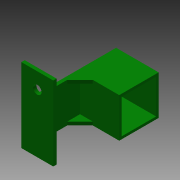
# Autodesk Inventor part: cameraMount
Saved by Autodesk Inventor 2014 (Build 180170000, 170)
## iProperties
Created: 2014-03-23
Part Number: cameraMount
Material: Generic
Document SubType Name: Modeling
Designer: jferner
Density: 1 g/cm^3
Appearance: Dark Green
Author: jferner
Autodesk Inventor part; units mm, degrees
ref_plane "YZ Plane" through (0, 0, 0) normal (1, 0, 0) x (0, 1, 0)
ref_plane "XZ Plane" through (0, 0, 0) normal (0, 1, 0) x (-1, 0, 0)
ref_plane "XY Plane" through (0, 0, 0) normal (0, 0, 1) x (1, 0, 0)
sketch "Sketch2" plane through (0, 0, 0) normal (1, 0, 0) x (0, 1, 0)
  line L0 (0, 0) -> (23.55, 0)
  line L1 (23.55, 0) -> (23.55, 23.55)
  line L2 (23.55, 23.55) -> (0, 23.55)
  line L3 (0, 23.55) -> (0, 0)
  line L4 (1.5, 1.5) -> (22.05, 1.5)
  line L5 (22.05, 1.5) -> (22.05, 22.05)
  line L6 (22.05, 22.05) -> (1.5, 22.05)
  line L7 (1.5, 22.05) -> (1.5, 1.5)
  dimension "d0" = 1.5
  dimension "d1" = 1.5
  dimension "d2" = 1.5
  dimension "d3" = 1.5
  dimension "d4" = 20.55
  dimension "d5" = 20.55
  dimension "widthSqAlum" = 23.55
  constraints: 16 end point, 4 parallel, 2 horizontal, 2 perpendicular
  measures "d0" distance between parallel lines of L3 L7
  measures "d1" distance between parallel lines of L0 L4
  measures "d2" distance between parallel lines of L1 L5
  measures "d3" distance between parallel lines of L2 L6
  measures "d4" distance between parallel lines of L6 L4
  measures "d5" distance of L4.start L4.end
  measures "widthSqAlum" distance of L1.end L2.end
extrude "Extrusion1" add sketch "Sketch2" along normal blind 25.4
sketch "Sketch3" plane through (0, 0, 0) normal (-1, 0, 0) x (0, 0, 1)
  line L0 (23.55, 0) -> (56.5781, 0)
  line L1 (56.5781, 0) -> (56.5781, 23.55)
  line L2 (56.5781, 23.55) -> (23.55, 23.55)
  line L3 (23.55, 23.55) -> (23.55, 0)
  dimension "d8" = 33.0281
  dimension "d9" = 23.55
  constraints: 8 end point, 2 parallel, 1 horizontal, 1 perpendicular
  measures "d8" distance of L1.end L2.end
  measures "d9" distance of L0.end L1.end
extrude "Extrusion2" add sketch "Sketch3" against normal blind 2
sketch "Sketch6" plane through (0, 0, 56.5781) normal (0, 0, 1) x (1, 0, 0)
  line L0 (0, 0) -> (0, 23.55) projected
  line L1 (0, 0) -> (2, 0) projected
  line L2 (2, 23.55) -> (2, 0) projected
  line L3 (0, 23.55) -> (2, 23.55) projected
  line L4 (0, 0) -> (19.05, 0)
  line L5 (19.05, 0) -> (19.05, 44.45)
  line L6 (19.05, 44.45) -> (0, 44.45)
  line L7 (0, 44.45) -> (0, 0)
  dimension "d21" = 44.45
  dimension "d22" = 19.05
  constraints: 8 end point, 2 parallel, 1 horizontal, 1 perpendicular
  measures "d21" distance of L4.end L5.end
  measures "d22" distance of L5.end L6.end
extrude "Extrusion5" add sketch "Sketch6" against normal blind 2 contours L7 L6 L5 L4 L2 L3
sketch "Sketch7" plane through (0, 44.45, 56.5781) normal (0, 0, 1) x (1, 0, 0)
  line L0 (19.05, -44.45) -> (19.05, 0) projected
  line L1 (19.05, 0) -> (0, 0) projected
  circle A0 centre (9.525, -9.525) radius 2.54
  dimension "d25" = 5.08
  dimension "d26" = 9.525
  dimension "d27" = 9.525
  constraints: 1 centre point
  measures "d25" diameter of A0
  measures "d26" distance from line of L1 A0.centre
  measures "d27" distance from line of L0 A0.centre
extrude "Extrusion6" cut sketch "Sketch7" against normal up to next
sketch "Sketch10" plane through (0, 23.55, 0) normal (0, 1, 0) x (1, 0, 0)
  line L0 (2, -23.55) -> (2, -54.5781) projected
  line L1 (2, -23.55) -> (25.4, -23.55) projected
  line L2 (0, 0) -> (0, -54.5781) projected
  line L3 (2, -54.5781) -> (9.62, -54.5781)
  line L4 (9.62, -54.5781) -> (2, -46.9581)
  line L5 (2, -23.55) -> (9.62, -23.55)
  line L6 (2, -31.17) -> (9.62, -23.55)
  dimension "d30" = 7.62
  dimension "d31" = 45
  dimension "d32" = 7.62
  dimension "d33" = 45
  constraints: 8 end point, 3 point on line, 1 perpendicular
  measures "d30" distance of L0.start L5.end
  measures "d31" angle of L0 L6
  measures "d32" distance of L0.end L3.end
  measures "d33" angle of L0 L4
extrude "Extrusion8" add sketch "Sketch10" against normal blind 2
sketch "Sketch11" plane through (0, 0, 0) normal (0, -1, 0) x (1, 0, 0)
  line L0 (2, 23.55) -> (25.4, 23.55) projected
  line L1 (2, 54.5781) -> (2, 23.55) projected
  line L2 (19.05, 54.5781) -> (2, 54.5781) projected
  line L3 (2, 54.5781) -> (9.62, 54.5781)
  line L4 (9.62, 54.5781) -> (2, 46.9581)
  line L5 (2, 23.55) -> (9.62, 23.55)
  line L6 (9.62, 23.55) -> (2, 31.17)
  dimension "d44" = 45
  dimension "d45" = 45
  dimension "d46" = 7.62
  dimension "d47" = 7.62
  constraints: 8 end point, 4 point on line
  measures "d44" angle of L1 L4
  measures "d45" angle of L1 L6
  measures "d46" distance of L1.start L3.end
  measures "d47" distance of L0.start L5.end
extrude "Extrusion9" add sketch "Sketch11" against normal blind 2
equation "\"d0\" = wallThicknessSqAlum"
equation "\"d1\" = wallThicknessSqAlum"
equation "\"d2\" = wallThicknessSqAlum"
equation "\"d3\" = wallThicknessSqAlum"
equation "\"d4\" = sqAlumWidth + sqAlumTolerance"
equation "\"d5\" = sqAlumWidth + sqAlumTolerance"
equation "\"d8\" = -cameraLensHeight + screwDistanceFromFront - wallThicknessSqAlum - 0.5 * sqAlumWidth"
equation "\"d9\" = widthSqAlum"
equation "\"d21\" = heightSqAlum + d22"
equation "\"d23\" = armWallThickness"
equation "\"d26\" = 0.5 * d22"
equation "\"d27\" = 0.5 * d22"
equation "\"d28\" = armWallThickness"
equation "\"d32\" = d30"
equation "\"d33\" = d31"
equation "\"d42\" = armWallThickness"
equation "\"d44\" = d31"
equation "\"d45\" = d31"
equation "\"d46\" = d30"
equation "\"d47\" = d30"
equation "\"d48\" = armWallThickness"
equation "\"sqAlumTolerance\" = 1.5"
equation "\"wallThicknessSqAlum\" = 1.5"
equation "\"sqAlumWidth\" = 19.05"
equation "\"cameraLensHeight\" = 31.75"
equation "\"screwDistanceFromFront\" = 75.803125"
equation "\"heightSqAlum\" = 25.4"
equation "\"armWallThickness\" = 2"
body "Solid1"
